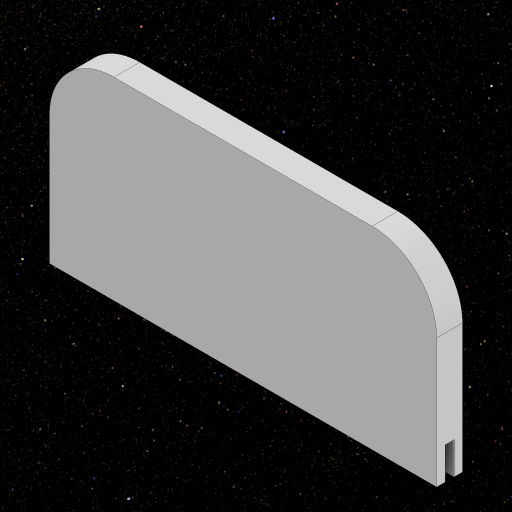
# Autodesk Inventor part: !caddy_wall
Saved by Autodesk Inventor 2024 (Build 280153000, 153)
## iProperties
Created: 2024-02-15
Part Number: !caddy_wall
Material: Generic
Document SubType Name: Modeling
Designer: Averey Ku
Density: 1 g/cm^3
Appearance: Default
Author: Averey Ku
Autodesk Inventor part; units mm, degrees
ref_plane "YZ Plane" through (0, 0, 0) normal (1, 0, 0) x (0, 1, 0)
ref_plane "XZ Plane" through (0, 0, 0) normal (0, 1, 0) x (-1, 0, 0)
ref_plane "XY Plane" through (0, 0, 0) normal (0, 0, 1) x (1, 0, 0)
sketch "Sketch1" plane through (0, 0, 0) normal (0, 0, 1) x (1, 0, 0)
  line L0 (0, 0) -> (76.2, 0)
  line L1 (76.2, 0) -> (76.2, 25.4)
  line L2 (63.5, 38.1) -> (12.7, 38.1)
  line L3 (0, 25.4) -> (0, 0)
  arc A0 (12.7, 38.1) -> (0, 25.4) centre (12.7, 25.4) ccw
  arc A1 (76.2, 25.4) -> (63.5, 38.1) centre (63.5, 25.4) ccw
  point P0 (76.2, 38.1)
  dimension "d0" = 76.2
  dimension "d1" = 38.1
  dimension "d2" = 12.7
  constraints: 8 end point, 4 point on circle, 4 tangent, 3 perpendicular, 2 centre point, 2 point on line, 1 equal radius, 1 horizontal
  measures "d0" distance of L0.start L0.end
  measures "d1" distance of L0.end point (76.2, 38.1)
  measures "d2" radius of A0
extrude "Extrusion1" add sketch "Sketch1" along normal blind 5.08
sketch "Sketch2" plane through (76.2, 0, 0) normal (1, 0, 0) x (0, 0, -1)
  line L0 (0, 0) -> (-5.08, 0) projected
  line L1 (-1.651, 0) -> (-1.651, 6.35)
  line L2 (-1.651, 6.35) -> (-3.429, 6.35)
  line L3 (-3.429, 6.35) -> (-3.429, 0)
  line L4 (-3.429, 0) -> (-1.651, 0)
  dimension "d5" = 6.35
  dimension "d6" = 1.778
  constraints: 8 end point, 2 perpendicular, 2 point on line, 1 horizontal
  measures "d5" distance of L1.start L1.end
  measures "d6" distance of L1.end L2.end
extrude "Extrusion2" cut sketch "Sketch2" against normal blind 101.6
body "Solid1"
